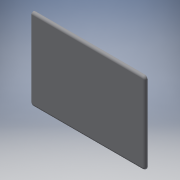
# Autodesk Inventor part: lid
Saved by Autodesk Inventor 2019 (Build 230136000, 136)
## iProperties
Created: 2021-11-14
Part Number: lid
Material: Generic
Document SubType Name: Modeling
Designer: Tiarnan Rice
Density: 1 g/cm^3
Appearance: Default
Author: Tiarnan Rice
Autodesk Inventor part; units mm, degrees
ref_plane "YZ Plane" through (0, 0, 0) normal (1, 0, 0) x (0, 1, 0)
ref_plane "XZ Plane" through (0, 0, 0) normal (0, 1, 0) x (-1, 0, 0)
ref_plane "XY Plane" through (0, 0, 0) normal (0, 0, 1) x (1, 0, 0)
sketch "Sketch1" plane through (0, 0, 0) normal (0, 0, 1) x (1, 0, 0)
  line L0 (11.04, 46.72) -> (11.04, 49.72) projected
  line L1 (11.04, 49.72) -> (-66.54, 49.72) projected
  arc A0 (-66.54, 49.72) -> (-70.04, 46.22) centre (-66.54, 46.22) ccw projected
  line L2 (-70.04, 46.22) -> (-70.04, -46.22) projected
  arc A1 (-70.04, -46.22) -> (-66.54, -49.72) centre (-66.54, -46.22) ccw projected
  line L3 (-66.54, -49.72) -> (11.04, -49.72) projected
  line L4 (11.04, -49.72) -> (11.04, -46.72) projected
  line L5 (11.04, -46.72) -> (-63.54, -46.72) projected
  arc A2 (-67.04, -43.22) -> (-63.54, -46.72) centre (-63.54, -43.22) ccw projected
  line L6 (-67.04, -43.22) -> (-67.04, 43.22) projected
  arc A3 (-63.54, 46.72) -> (-67.04, 43.22) centre (-63.54, 43.22) ccw projected
  line L7 (-63.54, 46.72) -> (11.04, 46.72) projected
  line L8 (11.04, 49.72) -> (14.54, 49.72) projected
  line L9 (14.54, 49.72) -> (57.54, 49.72) projected
  line L10 (57.54, 49.72) -> (61.04, 49.72) projected
  line L11 (61.04, 49.72) -> (61.04, 46.72) projected
  line L12 (61.04, 46.72) -> (63.54, 46.72) projected
  arc A4 (67.04, 43.22) -> (63.54, 46.72) centre (63.54, 43.22) ccw projected
  line L13 (67.04, 43.22) -> (67.04, -43.22) projected
  arc A5 (63.54, -46.72) -> (67.04, -43.22) centre (63.54, -43.22) ccw projected
  line L14 (63.54, -46.72) -> (61.04, -46.72) projected
  line L15 (61.04, -46.72) -> (61.04, -49.72) projected
  line L16 (61.04, -49.72) -> (66.54, -49.72) projected
  arc A6 (66.54, -49.72) -> (70.04, -46.22) centre (66.54, -46.22) ccw projected
  line L17 (70.04, -46.22) -> (70.04, 46.22) projected
  arc A7 (70.04, 46.22) -> (66.54, 49.72) centre (66.54, 46.22) ccw projected
  line L18 (66.54, 49.72) -> (61.04, 49.72) projected
  line L19 (57.54, -49.72) -> (61.04, -49.72) projected
  line L20 (57.54, -49.72) -> (14.54, -49.72) projected
  line L21 (11.04, -49.72) -> (14.54, -49.72) projected
  line L22 (14.54, 46.72) -> (11.04, 46.72) projected
  line L23 (57.54, 46.72) -> (14.54, 46.72) projected
  line L24 (61.04, 46.72) -> (57.54, 46.72) projected
  line L25 (61.04, -46.72) -> (57.54, -46.72) projected
  line L26 (14.54, -46.72) -> (57.54, -46.72) projected
  line L27 (14.54, -46.72) -> (11.04, -46.72) projected
  line L28 (-63.54, 46.72) -> (61.04, 46.72)
  line L29 (67.04, 43.22) -> (67.04, -43.22)
  line L30 (63.54, -46.72) -> (-63.54, -46.72)
  line L31 (-67.04, -43.22) -> (-67.04, 43.22)
  arc A8 (-63.54, 46.72) -> (-67.04, 43.22) centre (-63.54, 43.22) ccw
  line L32 (61.04, 46.72) -> (63.54, 46.72)
  arc A9 (67.04, 43.22) -> (63.54, 46.72) centre (63.54, 43.22) ccw
  arc A10 (63.54, -46.72) -> (67.04, -43.22) centre (63.54, -43.22) ccw
  arc A11 (-67.04, -43.22) -> (-63.54, -46.72) centre (-63.54, -43.22) ccw
  line L33 (61.04, 46.32) -> (-63.54, 46.32)
  arc A12 (-63.54, 46.32) -> (-66.64, 43.22) centre (-63.54, 43.22) ccw
  line L34 (-66.64, 43.22) -> (-66.64, -43.22)
  arc A13 (-66.64, -43.22) -> (-63.54, -46.32) centre (-63.54, -43.22) ccw
  line L35 (-63.54, -46.32) -> (63.54, -46.32)
  arc A14 (63.54, -46.32) -> (66.64, -43.22) centre (63.54, -43.22) ccw
  line L36 (66.64, -43.22) -> (66.64, 43.22)
  arc A15 (66.64, 43.22) -> (63.54, 46.32) centre (63.54, 43.22) ccw
  line L37 (63.54, 46.32) -> (61.04, 46.32)
  point P0 (0, 0)
  dimension "d0" = 0.4
  constraints: 20 end point, 16 point on circle, 8 centre point, 4 collinear, 4 tangent, 3 concentric, 2 perpendicular, 8 other
  measures "d0" distance between parallel lines of L28 L33
extrude "Extrusion1" add sketch "Sketch1" against normal blind 3 contours L37 A15 L36 A14 L35 A13 L34 A12 L33
sketch "Sketch2" plane through (0, 0, 0) normal (0, 0, 1) x (1, 0, 0)
  line L0 (11.04, 49.72) -> (-66.54, 49.72) projected
  arc A0 (-66.54, 49.72) -> (-70.04, 46.22) centre (-66.54, 46.22) ccw projected
  line L1 (-70.04, 46.22) -> (-70.04, -46.22) projected
  arc A1 (-70.04, -46.22) -> (-66.54, -49.72) centre (-66.54, -46.22) ccw projected
  line L2 (-66.54, -49.72) -> (11.04, -49.72) projected
  line L3 (11.04, -49.72) -> (14.54, -49.72) projected
  line L4 (57.54, -49.72) -> (14.54, -49.72) projected
  line L5 (57.54, -49.72) -> (61.04, -49.72) projected
  line L6 (61.04, -49.72) -> (66.54, -49.72) projected
  arc A2 (66.54, -49.72) -> (70.04, -46.22) centre (66.54, -46.22) ccw projected
  line L7 (70.04, -46.22) -> (70.04, 46.22) projected
  arc A3 (70.04, 46.22) -> (66.54, 49.72) centre (66.54, 46.22) ccw projected
  line L8 (66.54, 49.72) -> (61.04, 49.72) projected
  line L9 (57.54, 49.72) -> (61.04, 49.72) projected
  line L10 (14.54, 49.72) -> (57.54, 49.72) projected
  line L11 (11.04, 49.72) -> (14.54, 49.72) projected
  point P0 (0, 0)
extrude "Extrusion2" add sketch "Sketch2" along normal blind 3
fillet "Fillet1" radius 3 8 edges at (-69.0149, 48.6949, 3) (-70.04, 0, 3) (-69.0149, -48.6949, 3) (0, -49.72, 3) (69.0149, -48.6949, 3) (70.04, 0, 3) (69.0149, 48.6949, 3) (0, 49.72, 3)
body "Solid1"
